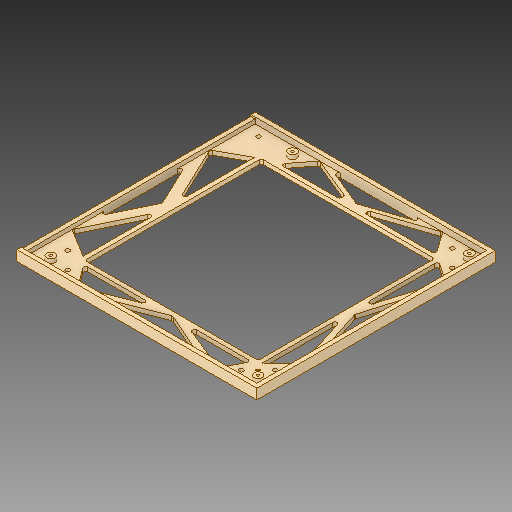
# Autodesk Inventor part: jetsonHolder
Saved by Autodesk Inventor 2018 (Build 220112000, 112)
## iProperties
Created: 2018-06-02
Part Number: jetsonHolder
Material: Polyethylene, High Density
Document SubType Name: Modeling
Designer: Cole Tucker
Density: 0.952 g/cm^3
Appearance: Smooth - Off-White
Mass: 35.3598 g
Surface Area: 322.769 cm^2
Volume: 37.1427 cm^3
Author: Cole Tucker
Autodesk Inventor part; units mm, degrees
ref_plane "YZ Plane" through (0, 0, 0) normal (1, 0, 0) x (0, 1, 0)
ref_plane "XZ Plane" through (0, 0, 0) normal (0, 1, 0) x (-1, 0, 0)
ref_plane "XY Plane" through (0, 0, 0) normal (0, 0, 1) x (1, 0, 0)
sketch "Sketch1" plane through (0, 0, 0) normal (0, 1, 0) x (-1, 0, 0)
  line L0 (0, 0) -> (-6, 0) construction
  line L1 (-6, 0) -> (-6, 7) construction
  line L2 (-6, 7) -> (0, 7) construction
  line L3 (0, 7) -> (0, 0) construction
  line L4 (0, 0) -> (155.25, 0) construction
  line L5 (155.25, 0) -> (167.25, 0) construction
  line L6 (167.25, 0) -> (167.25, 7) construction
  line L7 (167.25, 7) -> (155.25, 7) construction
  line L8 (155.25, 7) -> (155.25, 0) construction
  line L9 (0, 0) -> (0, -158) construction
  line L10 (0, -158) -> (-6, -158) construction
  line L11 (-6, -158) -> (-6, -165) construction
  line L12 (-6, -165) -> (0, -165) construction
  line L13 (0, -165) -> (0, -158) construction
  line L14 (0, -158) -> (132.28, -158) construction
  line L15 (132.28, -158) -> (167.25, -158) construction
  line L16 (167.25, -158) -> (167.25, -165) construction
  line L17 (167.25, -165) -> (132.28, -165) construction
  line L18 (132.28, -165) -> (132.28, -158) construction
  line L19 (167.25, 0) -> (167.25, -158) construction
  line L20 (-6, 7) -> (167.25, 7)
  line L21 (167.25, 7) -> (167.25, -165)
  line L22 (167.25, -165) -> (-6, -165)
  line L23 (-6, -165) -> (-6, 7)
  dimension "d0" = 6
  dimension "d1" = 7
  dimension "d2" = 155.25
  dimension "d4" = 7
  dimension "d5" = 158
  dimension "d6" = 6
  dimension "d7" = 7
  dimension "d8" = 132.28
  dimension "d45" = 7
  dimension "d46" = 12
  constraints: 48 end point, 10 parallel, 7 horizontal, 5 perpendicular, 4 coincident, 2 vertical
  measures "d0" distance of L1.end L2.end
  measures "d1" distance of L0.end L1.end
  measures "d2" distance of L0.start L4.end
  measures "d4" distance of L6.end L5.end
  measures "d5" distance of L0.start L9.end
  measures "d6" distance of L12.end L11.end
  measures "d7" distance of L10.end L11.end
  measures "d8" distance of L14.start L14.end
  measures "d45" distance of L17.end L14.end
  measures "d46" distance of L6.end L7.end
extrude "Extrusion1" add sketch "Sketch1" along normal blind 3.175
hole "Hole1" at (-155.25, 0, 0) at (0, 0, 0) at (0, 0, -158) at (-132.28, 0, -158) direction (0, 1, 0) diameter 2.032 depth 25.4 tip angle 118
sketch "Sketch2" plane through (0, 0, 0) normal (0, -1, 0) x (1, 0, 0)
  circle A0 centre (0, 0) radius 1.016 construction
  line L0 (0, 0) -> (-12.7, 0) construction
  line L1 (-12.7, 0) -> (-12.7, -12.7) construction
  line L2 (-12.7, -12.7) -> (0, -12.7) construction
  line L3 (0, -12.7) -> (0, 0) construction
  circle A1 centre (-155.25, 0) radius 1.016 construction
  line L4 (-155.25, 0) -> (-155.25, -157.48) construction
  line L5 (-155.25, -157.48) -> (-142.55, -157.48) construction
  line L6 (-142.55, -157.48) -> (-142.55, -144.78) construction
  line L7 (-142.55, -144.78) -> (-155.25, -144.78) construction
  line L8 (-155.25, -144.78) -> (-155.25, -157.48) construction
  line L9 (-142.55, -144.78) -> (-12.7, -144.78)
  line L10 (-12.7, -144.78) -> (-12.7, -12.7)
  line L11 (-12.7, -12.7) -> (-142.55, -12.7)
  line L12 (-142.55, -12.7) -> (-142.55, -144.78)
  dimension "d18" = 12.7
  dimension "d19" = 12.7
  dimension "d20" = 12.7
  dimension "d21" = 12.7
  constraints: 26 end point, 6 parallel, 3 horizontal, 3 perpendicular, 1 vertical
  measures "d18" distance of L2.end L1.end
  measures "d19" distance of L1.end L0.end
  measures "d20" distance of L7.end L6.end
  measures "d21" distance of L6.end L5.end
extrude "Extrusion2" cut sketch "Sketch2" against normal blind 3.175
sketch "Sketch3" plane through (0, 0, 0) normal (0, -1, 0) x (1, 0, 0)
  line L0 (-12.7, -12.7) -> (-142.55, -12.7) projected
  line L1 (-142.55, -12.7) -> (-142.55, -144.78) projected
  line L2 (-142.55, -144.78) -> (-12.7, -144.78) projected
  line L3 (-12.7, -144.78) -> (-12.7, -12.7) projected
  line L4 (-167.25, 7) -> (6, 7) projected
  line L5 (6, 7) -> (6, -165) projected
  line L6 (6, -165) -> (-167.25, -165) projected
  line L7 (-167.25, -165) -> (-167.25, 7) projected
  line L8 (-12.7, -12.7) -> (-142.55, -12.7) projected
  line L9 (-142.55, -12.7) -> (-142.55, -144.78) projected
  line L10 (-142.55, -144.78) -> (-12.7, -144.78) projected
  line L11 (-12.7, -144.78) -> (-12.7, -12.7) projected
  line L12 (-167.25, 7) -> (6, 7) projected
  line L13 (6, 7) -> (6, -165) projected
  line L14 (6, -165) -> (-167.25, -165) projected
  line L15 (-167.25, -165) -> (-167.25, 7) projected
  line L16 (-167.25, -165) -> (-170.425, -165) construction
  line L17 (-170.425, -165) -> (-170.425, -168.175) construction
  line L18 (-170.425, -168.175) -> (-167.25, -168.175) construction
  line L19 (-167.25, -168.175) -> (-167.25, -165) construction
  line L20 (-167.25, 7) -> (6, 7) construction
  line L21 (6, 7) -> (9.175, 7) construction
  line L22 (9.175, 7) -> (9.175, 10.175) construction
  line L23 (9.175, 10.175) -> (6, 10.175) construction
  line L24 (6, 10.175) -> (6, 7) construction
  line L25 (6, 7) -> (-167.25, 7)
  line L26 (-167.25, 7) -> (-167.25, -165)
  line L27 (-167.25, -165) -> (6, -165)
  line L28 (6, -165) -> (6, 7)
  line L29 (9.175, 10.175) -> (-170.425, 10.175)
  line L30 (-170.425, 10.175) -> (-170.425, -168.175)
  line L31 (-170.425, -168.175) -> (9.175, -168.175)
  line L32 (9.175, -168.175) -> (9.175, 10.175)
  dimension "d47" = 3.175
  dimension "d48" = 3.175
  dimension "d49" = 3.175
  dimension "d50" = 3.175
  constraints: 32 end point, 8 parallel, 4 horizontal, 4 perpendicular
  measures "d47" distance of L18.end L17.end
  measures "d48" distance of L17.end L16.end
  measures "d49" distance of L23.end L22.end
  measures "d50" distance of L22.end L21.end
sketch "Sketch4" plane through (0, 3.175, 0) normal (0, 1, 0) x (1, 0, 0)
  line L0 (-12.7, 144.78) -> (-12.7, 12.7) construction
  circle A0 centre (0, 0) radius 1.016 construction
  line L1 (-12.7, 12.7) -> (0, 0) construction
  line L2 (-6.35, 6.35) -> (-7.4815, 5.2185) construction
  line L3 (-7.4815, 5.2185) -> (-5.2364, 7.4636)
  line L4 (-6.35, 6.35) -> (-4.5539, 4.5539) construction
  line L5 (-4.5539, 4.5539) -> (-7.4815, 5.2185)
  line L6 (-4.5539, 4.5539) -> (-5.2364, 7.4636)
  dimension "d32" = 1.6002
  dimension "d33" = 3.175
  dimension "d34" = 2.54
  constraints: 12 end point, 2 point on line, 1 midpoint
  measures "d32" distance of L2.start L2.end
  measures "d33" distance of L2.end L3.end
  measures "d34" distance of L2.start L4.end
extrude "Extrusion4" add sketch "Sketch4" along normal blind 0.254
sketch "Sketch5" plane through (0, 3.175, 0) normal (0, 1, 0) x (1, 0, 0)
  circle A0 centre (0, 0) radius 1.016 projected
  circle A1 centre (0, 0) radius 3.175
  circle A2 centre (0, 158) radius 1.016 projected
  circle A3 centre (0, 158) radius 3.175
  circle A4 centre (-132.28, 158) radius 1.016 projected
  circle A5 centre (-132.28, 158) radius 3.175
  line L0 (-5.2364, 7.4636) -> (-4.5539, 4.5539) projected
  line L1 (-4.5539, 4.5539) -> (-7.4815, 5.2185) projected
  line L2 (-7.4815, 5.2185) -> (-5.2364, 7.4636) projected
  line L3 (-12.7, 12.7) -> (-142.55, 12.7) projected
  line L4 (-142.55, 12.7) -> (-142.55, 144.78) projected
  line L5 (-142.55, 144.78) -> (-12.7, 144.78) projected
  line L6 (-12.7, 144.78) -> (-12.7, 12.7) projected
  circle A6 centre (0, 158) radius 1.016 projected
  circle A7 centre (-155.25, 0) radius 1.016 projected
  circle A8 centre (0, 0) radius 1.016 projected
  circle A9 centre (-132.28, 158) radius 1.016 projected
  circle A10 centre (-155.25, 0) radius 1.016 projected
  circle A11 centre (-155.25, 0) radius 3.175
  dimension "d37" = 6.35
  dimension "d38" = 6.35
  dimension "d39" = 6.35
  dimension "d40" = 6.35
  constraints: 4 centre point, 4 coincident
  measures "d37" diameter of A1
  measures "d38" diameter of A3
  measures "d39" diameter of A5
  measures "d40" diameter of A11
extrude "Extrusion5" add sketch "Sketch5" along normal blind 3.175 contours A1 | A3 | A5 | A11
extrude "Extrusion6" add sketch "Sketch3" against normal blind 7.62 contours L32 L31 L30 L29
sketch "Sketch6" plane through (0, 7.62, 0) normal (0, 1, 0) x (1, 0, 0)
  line L0 (-167.25, 165) -> (-167.25, -7) projected
  line L1 (-170.425, 168.175) -> (-170.425, -10.175) projected
  line L2 (-167.25, -7) -> (-170.425, -7)
  line L3 (-170.425, -7) -> (-170.425, 164.9313)
  line L4 (-170.425, 164.9313) -> (-167.25, 164.9313)
  line L5 (-167.25, 164.9313) -> (-167.25, -7)
  point P0 (0, 0)
  constraints: 8 end point, 2 parallel, 1 horizontal, 1 perpendicular, 1 point on line
extrude "Extrusion7" cut sketch "Sketch6" against normal up to surface (1.27 mm away)
sketch "Sketch7" plane through (0, 3.175, 0) normal (0, 1, 0) x (1, 0, 0)
  circle A0 centre (0, 0) radius 1.016 projected
  line L0 (0, 0) -> (-12.7, 0)
  line L1 (0, 0) -> (0, 12.7)
  circle A1 centre (0, 158) radius 1.016 projected
  line L2 (0, 158) -> (-12.7, 158)
  line L3 (0, 158) -> (0, 145.3)
  circle A2 centre (-132.28, 158) radius 1.016 projected
  line L4 (-132.28, 158) -> (-144.98, 158)
  line L5 (-144.98, 158) -> (-157.68, 158)
  circle A3 centre (-155.25, 0) radius 1.016 projected
  line L6 (-155.25, 0) -> (-142.55, 0)
  line L7 (-155.25, 0) -> (-155.25, 12.7)
  dimension "d53" = 12.7
  dimension "d54" = 12.7
  dimension "d55" = 12.7
  dimension "d56" = 12.7
  dimension "d57" = 12.7
  dimension "d58" = 12.7
  dimension "d59" = 12.7
  dimension "d60" = 12.7
  constraints: 16 end point, 7 coincident, 4 horizontal, 2 perpendicular, 1 point on line, 1 vertical
  measures "d53" distance of L0.start L0.end
  measures "d54" distance of L0.start L1.end
  measures "d55" distance of L2.start L2.end
  measures "d56" distance of L2.start L3.end
  measures "d57" distance of L4.start L4.end
  measures "d58" distance of L4.end L5.end
  measures "d59" distance of L6.start L6.end
  measures "d60" distance of L6.start L7.end
hole "Hole2" at (-12.7, 3.175, 0) at (0, 3.175, -12.7) at (0, 3.175, -145.3) at (-12.7, 3.175, -158) at (-157.68, 3.175, -158) at (-142.55, 3.175, 0) at (-155.25, 3.175, -12.7) direction (0, -1, 0) diameter 3.175 depth 25.4 tip angle 118
sketch "Sketch8" plane through (0, 3.175, 0) normal (0, 1, 0) x (1, 0, 0)
  line L0 (-142.55, 12.7) -> (-12.7, 12.7) projected
  line L1 (-85.7322, 9.525) -> (-127.9282, -7)
  line L2 (-167.25, -7) -> (6, -7) projected
  line L3 (-142.55, 12.7) -> (-142.55, 144.78) projected
  line L4 (-127.9282, -7) -> (-140.1934, 9.525)
  line L5 (-142.55, 12.7) -> (-142.55, 9.525)
  line L6 (-142.55, 9.525) -> (-12.7, 9.525)
  line L7 (-14.3736, 9.525) -> (-23.0843, -7)
  line L8 (-23.0843, -7) -> (-63.6157, 9.525)
  line L9 (-115.7057, -7) -> (-73.5098, 9.525)
  line L10 (-35.8918, -7) -> (-73.5098, 9.525)
  line L11 (-35.8918, -7) -> (-115.7057, -7)
  point P0 (0, 0)
  dimension "d68" = 3.175
  constraints: 18 end point, 9 point on line, 3 parallel, 1 perpendicular
  measures "d68" distance of L0.start L5.end
extrude "Extrusion8" cut sketch "Sketch8" against normal blind 25.4 contours L1 L4 L6 | L10 L2 L9 | L6 L7 L8
sketch "Sketch9" plane through (0, 3.175, 0) normal (0, 1, 0) x (1, 0, 0)
  line L0 (-142.55, 144.78) -> (-142.55, 12.7) projected
  line L1 (-145.725, 14.6568) -> (-167.25, 27.9229)
  line L2 (-167.25, 164.9313) -> (-167.25, -7) projected
  line L3 (-12.7, 12.7) -> (-142.55, 12.7) projected
  line L4 (-142.55, 12.7) -> (-145.725, 12.7)
  line L5 (-145.725, 12.7) -> (-145.725, 144.78)
  line L6 (-12.7, 144.78) -> (-142.55, 144.78) projected
  line L7 (-145.725, 143.0191) -> (-167.25, 131.0808)
  line L8 (-167.25, 131.0808) -> (-145.725, 85.468)
  line L9 (-145.725, 72.2078) -> (-167.25, 27.9229)
  line L10 (-167.25, 44.387) -> (-150.5525, 78.74)
  line L11 (-150.5525, 78.74) -> (-167.25, 114.123)
  line L12 (-167.25, 44.387) -> (-167.25, 114.123)
  point P0 (0, 0)
  dimension "d71" = 3.175
  constraints: 18 end point, 8 point on line, 2 collinear, 2 parallel, 1 perpendicular
  measures "d71" distance of L0.end L4.end
extrude "Extrusion9" cut sketch "Sketch9" against normal blind 25.4 contours L1 L9 L5 | L2 L11 L10 | L8 L7 L5
sketch "Sketch10" plane through (0, 3.175, 0) normal (0, 1, 0) x (1, 0, 0)
  line L0 (-12.7, 144.78) -> (-142.55, 144.78) projected
  line L1 (-142.55, 144.78) -> (-142.55, 147.955)
  line L2 (-142.55, 147.955) -> (-12.7, 147.955)
  line L3 (-132.28, 147.955) -> (-119.0842, 165)
  line L4 (6, 165) -> (-167.25, 165) projected
  line L5 (-14.9055, 147.955) -> (-26.7455, 165)
  line L6 (-26.7455, 165) -> (-77.625, 147.955)
  line L7 (-77.625, 147.955) -> (-119.0842, 165)
  line L8 (-77.625, 147.955) -> (-77.625, 151.13)
  line L9 (-77.625, 151.13) -> (-111.3615, 165)
  line L10 (-77.625, 151.13) -> (-36.2229, 165)
  line L11 (-36.2229, 165) -> (-111.3615, 165)
  line L12 (-87.1024, 147.955) -> (-87.1024, 151.8514)
  line L13 (-68.3341, 147.955) -> (-68.3341, 151.0675)
  point P0 (0, 0)
  dimension "d74" = 3.175
  dimension "d75" = 3.175
  constraints: 24 end point, 9 point on line, 2 parallel, 2 perpendicular, 1 collinear, 1 midpoint, 1 vertical
  measures "d74" distance of L0.end L1.end
  measures "d75" distance of L6.end L8.end
extrude "Extrusion11" cut sketch "Sketch10" against normal blind 25.4 contours L3 L7 L12 L2 | L4 L10 L9 | L13 L6 L5 L2
sketch "Sketch11" plane through (0, 3.175, 0) normal (0, 1, 0) x (1, 0, 0)
  line L0 (-12.7, 12.7) -> (-142.55, 12.7) projected
  line L1 (-12.7, 12.7) -> (-9.525, 12.7)
  line L2 (-9.525, 12.7) -> (-9.525, 144.78)
  line L3 (-9.525, 144.78) -> (6, 134.0466)
  line L4 (6, -7) -> (6, 165) projected
  line L5 (-9.525, 12.7) -> (6, 26.829)
  line L6 (-9.525, 78.74) -> (-9.525, 75.565)
  line L7 (-9.525, 75.565) -> (6, 26.829)
  line L8 (-9.525, 78.74) -> (-9.525, 81.915)
  line L9 (-9.525, 81.915) -> (6, 134.0466)
  line L10 (-9.525, 78.74) -> (-6.35, 78.74)
  line L11 (-6.35, 78.74) -> (6, 39.9709)
  line L12 (-6.35, 78.74) -> (6, 120.2103)
  line L13 (6, 120.2103) -> (6, 39.9709)
  point P0 (0, 0)
  dimension "d80" = 3.175
  dimension "d81" = 3.175
  dimension "d82" = 3.175
  dimension "d83" = 3.175
  constraints: 24 end point, 6 point on line, 2 horizontal, 2 perpendicular, 1 midpoint
  measures "d80" distance of L0.start L1.end
  measures "d81" distance of L6.start L6.end
  measures "d82" distance of L6.start L8.end
  measures "d83" distance of L6.start L10.end
extrude "Extrusion12" cut sketch "Sketch11" against normal blind 25.4 contours L2 L7 L5 | L11 L12 L4 | L2 L3 L9
fillet "Fillet1" radius 1.6002 39 edges at (-68.3341, 1.5875, -151.0675) (-68.3341, 1.5875, -147.955) (-77.625, 1.5875, -151.13) (-87.1024, 1.5875, -151.8514) (-26.7455, 1.5875, -165) (-14.9055, 1.5875, -147.955) (-87.1024, 1.5875, -147.955) (-119.0842, 1.5875, -165) (-132.28, 1.5875, -147.955) (-167.25, 1.5875, -131.0808) (-36.2229, 1.5875, -165) (-111.3615, 1.5875, -165) (-6.35, 1.5875, -78.74) (-167.25, 1.5875, -27.9229) (-167.25, 1.5875, -114.123) (-167.25, 1.5875, -44.387) (-150.5525, 1.5875, -78.74) (-142.55, 1.5875, -144.78) (-145.725, 1.5875, -72.2078) (-145.725, 1.5875, -85.468) (-85.7322, 1.5875, -9.525) (-73.5098, 1.5875, -9.525) (-63.6157, 1.5875, -9.525) (-14.3736, 1.5875, -9.525) (-12.7, 1.5875, -144.78) (-9.525, 1.5875, -144.78) (6, 1.5875, -134.0466) (-9.525, 1.5875, -81.915) (-9.525, 1.5875, -75.565) (6, 1.5875, -26.829) (6, 1.5875, -39.9709) (6, 1.5875, -120.2103) (-12.7, 1.5875, -12.7) (-142.55, 1.5875, -12.7) (-140.1934, 1.5875, -9.525) (-127.9282, 1.5875, 7) (-115.7057, 1.5875, 7) (-35.8918, 1.5875, 7) (-23.0843, 1.5875, 7)
equation "\"d4\" = d1"
equation "\"d6\" = d0"
equation "\"d7\" = d1"
equation "\"d45\" = d1"
body "Solid1"
